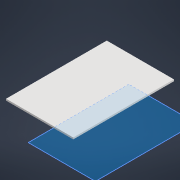
# Autodesk Inventor part: slide_panel
Saved by Autodesk Inventor 2021 (Build 250183000, 183)
## iProperties
Created: 2023-03-30
Part Number: slide_panel
Material: 一般
Document SubType Name: Modeling
Designer: casey
Density: 1 g/cm^3
Appearance: 既定
Author: casey
Autodesk Inventor part; units mm, degrees
ref_plane "YZ Plane" through (0, 0, 0) normal (1, 0, 0) x (0, 1, 0)
ref_plane "XZ Plane" through (0, 0, 0) normal (0, 1, 0) x (-1, 0, 0)
ref_plane "XY Plane" through (0, 0, 0) normal (0, 0, 1) x (1, 0, 0)
sketch "スケッチ1" plane through (0, 0, 0) normal (0, 1, 0) x (-1, 0, 0)
  line L0 (0, 0) -> (160, 0)
  line L1 (160, 0) -> (160, -240)
  line L2 (160, -240) -> (0, -240)
  line L3 (0, -240) -> (0, 0)
  dimension "d0" = 160
  dimension "d1" = 240
  constraints: 8 end point, 2 parallel, 1 horizontal, 1 perpendicular
  measures "d0" distance of L1.end L2.end
  measures "d1" distance of L0.end L1.end
extrude "押し出し1" add sketch "スケッチ1" along normal blind 4
sketch "スケッチ3" plane through (0, 4, 0) normal (0, 1, 0) x (1, 0, 0)
  line L0 (-160, 240) -> (-160, 0) projected
  line L1 (-160, 0) -> (0, 0) projected
  line L2 (0, 240) -> (-160, 240) projected
  point P0 (-153, 7)
  point P1 (-153, 233)
  point P2 (-153, 120)
  point P3 (-160, 120)
  dimension "d11" = 7
  dimension "d12" = 7
  dimension "d13" = 7
  dimension "d14" = 7
  dimension "d15" = 7
  dimension "d16" = 0
  constraints: 1 midpoint
  measures "d11" distance from line of L0 point (-153, 7)
  measures "d12" distance from line of point (-153, 7) L1
  measures "d13" distance from line of L0 point (-153, 233)
  measures "d14" distance from line of point (-153, 233) L2
  measures "d15" distance from line of L0 point (-153, 120)
  measures "d16" vertical distance of point (-153, 120) point (-160, 120)
hole "穴1" at (-153, 4, -7) at (-153, 4, -233) at (-153, 4, -120) direction (0, -1, 0) diameter 3.5 end through all
sketch "スケッチ4" plane through (0, 0, 0) normal (0, -1, 0) x (1, 0, 0)
  point P0 (0, 0)
